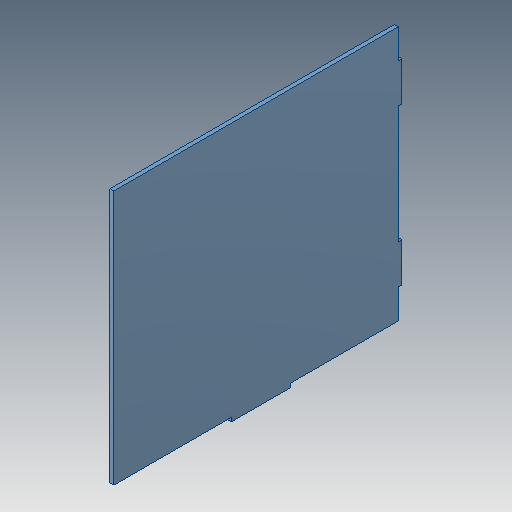
# Autodesk Inventor part: sidePlate
Saved by Autodesk Inventor 2018 (Build 220112000, 112)
## iProperties
Created: 2017-11-16
Part Number: sidePlate
Material: Aluminum 6061
Document SubType Name: Modeling
Designer: Udara Wanasinghe
Density: 2.7 g/cm^3
Appearance: Aluminum - Flat(1)
Mass: 102.562 g
Surface Area: 391.233 cm^2
Volume: 37.986 cm^3
Author: Udara Wanasinghe
Autodesk Inventor part; units mm, degrees
ref_plane "YZ Plane" through (0, 0, 0) normal (1, 0, 0) x (0, 1, 0)
sketch "Sketch1" plane through (0, 0, 0) normal (0, 1, 0) x (-1, 0, 0)
  line L0 (1, 75) -> (-1, 75)
  line L1 (-1, 75) -> (-1, -70.101)
  line L2 (-1, -75) -> (0, -75) construction
  line L3 (1, -75) -> (1, -70.101) construction
  line L4 (0, 75) -> (0, -75) construction
  arc A0 (1, -70.101) -> (-1, -70.101) centre (0, -75) ccw
  arc A1 (-1, -70.101) -> (1, -70.101) centre (0, -75) ccw construction
  line L5 (1, -70.101) -> (1, 75)
  line L6 (0, -75) -> (1, -75) construction
  line L7 (-1, -70.101) -> (-1, -75) construction
  point P0 (0, 0)
  point P1 (0, 0)
  dimension "d0" = 2
  dimension "d1" = 150
  dimension "d18" = 10
  constraints: 16 end point, 6 parallel, 4 point on circle, 2 centre point, 2 coincident, 2 midpoint, 2 perpendicular, 1 horizontal
  measures "d0" distance of L3.start L2.start
  measures "d1" distance of L0.end L2.start
  measures "d18" diameter of A0
extrude "Extrusion1" add sketch "Sketch1" along normal blind 130
ref_plane "Work Plane2" through (0, 0, 0) normal (0, -1, 0) x (1, 0, 0)
sketch "Sketch2" plane through (0, 0, 0) normal (0, -1, 0) x (1, 0, 0)
  line L0 (1, 15) -> (-1, 15)
  line L1 (-1, 15) -> (-1, -15)
  line L2 (-1, -15) -> (1, -15)
  line L3 (1, -15) -> (1, 15)
  line L4 (0, 15) -> (0, -15) construction
  point P0 (0, 0)
  point P1 (0, 0)
  dimension "d5" = 2
  dimension "d6" = 30
  constraints: 10 end point, 3 midpoint, 2 parallel, 1 coincident, 1 horizontal, 1 perpendicular
  measures "d5" distance of L2.end L1.end
  measures "d6" distance of L1.end L0.end
extrude "Extrusion2" add sketch "Sketch2" along normal blind 2
ref_plane "Work Plane4" through (1, 0, -70) normal (0, 0, 1) x (1, 0, 0)
sketch "Sketch4" plane through (1, 0, -70) normal (0, 0, 1) x (1, 0, 0)
  line L0 (0, 115) -> (-2, 115)
  line L1 (-2, 115) -> (-2, 95)
  line L2 (-2, 95) -> (0, 95)
  line L3 (0, 95) -> (0, 115)
  line L4 (-1, 115) -> (-1, 95) construction
  line L5 (-1, 0) -> (-1, 130) construction
  line L6 (-2, 130) -> (0, 130) construction
  line L7 (-2, 35) -> (0, 35)
  line L8 (0, 35) -> (0, 15)
  line L9 (0, 15) -> (-2, 15)
  line L10 (-2, 15) -> (-2, 35)
  line L11 (-1, 35) -> (-1, 15) construction
  line L12 (-2, 0) -> (0, 0) construction
  dimension "d20" = 2
  dimension "d21" = 20
  dimension "d22" = 15
  dimension "d23" = 2
  dimension "d24" = 20
  dimension "d25" = 15
  constraints: 22 end point, 5 midpoint, 4 parallel, 2 collinear, 2 horizontal, 2 perpendicular
  measures "d20" distance of L2.end L1.end
  measures "d21" distance of L1.end L0.end
  measures "d22" distance between parallel lines of L0 L6
  measures "d23" distance of L8.end L9.end
  measures "d24" distance of L7.end L8.end
  measures "d25" distance between parallel lines of L12 L9
extrude "Extrusion4" add sketch "Sketch4" against normal blind 2
body "Solid1"
